Autodesk Inventor part; units mm, degrees
(part 3 of 3)
  line L665 (5.8356, -14.9844) -> (7.0568, -17.6988)
  line L666 (7.0568, -17.6988) -> (8.2692, -14.9844)
  line L667 (8.2692, -14.9844) -> (9.8603, -14.9844)
  line L668 (9.8603, -14.9844) -> (9.8603, -20.4844)
  spline S503 degree 2 poles (14.9057, -18.4119) (14.9057, -19.437) (13.787, -20.6137) (12.7663, -20.6137) knots 0 0 0 1 2 2 2
  spline S504 degree 2 poles (12.7663, -20.6137) (11.7501, -20.6137) (10.6225, -19.437) (10.6225, -18.4119) knots 0 0 0 1 2 2 2
  spline S505 degree 2 poles (10.6225, -18.4119) (10.6225, -17.3779) (11.7501, -16.2057) (12.7663, -16.2057) knots 0 0 0 1 2 2 2
  spline S506 degree 2 poles (12.7663, -16.2057) (13.7825, -16.2057) (14.9057, -17.3823) (14.9057, -18.4119) knots 0 0 0 1 2 2 2
  spline S507 degree 2 poles (13.582, -18.4208) (13.582, -18.0509) (13.4616, -17.5562) (13.3547, -17.4091) knots 0 0 0 1 2 2 2
  spline S508 degree 2 poles (13.3547, -17.4091) (13.2388, -17.2531) (12.9491, -17.1327) (12.7663, -17.1327) knots 0 0 0 1 2 2 2
  spline S509 degree 2 poles (12.7663, -17.1327) (12.588, -17.1327) (12.3073, -17.2397) (12.1914, -17.3912) knots 0 0 0 1 2 2 2
  spline S510 degree 2 poles (12.1914, -17.3912) (12.0799, -17.5339) (11.9462, -18.0375) (11.9462, -18.4208) knots 0 0 0 1 2 2 2
  spline S511 degree 2 poles (11.9462, -18.4208) (11.9462, -18.7997) (12.071, -19.2677) (12.1735, -19.4103) knots 0 0 0 1 2 2 2
  spline S512 degree 2 poles (12.1735, -19.4103) (12.2761, -19.5529) (12.588, -19.6866) (12.7752, -19.6866) knots 0 0 0 1 2 2 2
  spline S513 degree 2 poles (12.7752, -19.6866) (12.9312, -19.6866) (13.2521, -19.5529) (13.3502, -19.4192) knots 0 0 0 1 2 2 2
  spline S514 degree 2 poles (13.3502, -19.4192) (13.4616, -19.2632) (13.582, -18.813) (13.582, -18.4208) knots 0 0 0 1 2 2 2
  spline S515 degree 2 poles (16.8534, -20.5959) (16.3988, -20.5959) (15.5832, -20.3953) (15.3158, -20.2616) knots 0 0 0 1 2 2 2
  line L669 (15.3158, -20.2616) -> (15.3158, -19.1696)
  line L670 (15.3158, -19.1696) -> (15.4227, -19.1696)
  spline S516 degree 2 poles (15.4227, -19.1696) (15.5163, -19.2409) (15.7526, -19.4103) (15.962, -19.5039) knots 0 0 0 1 2 2 2
  spline S517 degree 2 poles (15.962, -19.5039) (16.1448, -19.5886) (16.5949, -19.7089) (16.8624, -19.7089) knots 0 0 0 1 2 2 2
  spline S518 degree 2 poles (16.8624, -19.7089) (17.1342, -19.7089) (17.5532, -19.5395) (17.5532, -19.3568) knots 0 0 0 1 2 2 2
  spline S519 degree 2 poles (17.5532, -19.3568) (17.5532, -19.2142) (17.3615, -19.0626) (17.0852, -19.0002) knots 0 0 0 1 2 2 2
  spline S520 degree 2 poles (17.0852, -19.0002) (16.9381, -18.9601) (16.488, -18.8754) (16.3141, -18.822) knots 0 0 0 1 2 2 2
  spline S521 degree 2 poles (16.3141, -18.822) (15.8239, -18.6704) (15.3336, -18.0776) (15.3336, -17.5918) knots 0 0 0 1 2 2 2
  spline S522 degree 2 poles (15.3336, -17.5918) (15.3336, -17.3155) (15.5876, -16.8252) (15.8372, -16.6335) knots 0 0 0 1 2 2 2
  spline S523 degree 2 poles (15.8372, -16.6335) (16.0824, -16.4463) (16.8089, -16.2235) (17.268, -16.2235) knots 0 0 0 1 2 2 2
  spline S524 degree 2 poles (17.268, -16.2235) (17.7047, -16.2235) (18.4357, -16.3973) (18.6853, -16.5177) knots 0 0 0 1 2 2 2
  line L671 (18.6853, -16.5177) -> (18.6853, -17.5695)
  line L672 (18.6853, -17.5695) -> (18.5828, -17.5695)
  spline S525 degree 2 poles (18.5828, -17.5695) (18.5159, -17.516) (18.2262, -17.3422) (18.0925, -17.2798) knots 0 0 0 1 2 2 2
  spline S526 degree 2 poles (18.0925, -17.2798) (17.9276, -17.2085) (17.5265, -17.1104) (17.317, -17.1104) knots 0 0 0 1 2 2 2
  spline S527 degree 2 poles (17.317, -17.1104) (17.0362, -17.1104) (16.6484, -17.3021) (16.6484, -17.4581) knots 0 0 0 1 2 2 2
  spline S528 degree 2 poles (16.6484, -17.4581) (16.6484, -17.6007) (16.8401, -17.7612) (17.161, -17.8414) knots 0 0 0 1 2 2 2
  spline S529 degree 2 poles (17.161, -17.8414) (17.3259, -17.8815) (17.7582, -17.9573) (17.9588, -18.0241) knots 0 0 0 1 2 2 2
  spline S530 degree 2 poles (17.9588, -18.0241) (18.4045, -18.1668) (18.868, -18.7239) (18.868, -19.1874) knots 0 0 0 1 2 2 2
  spline S531 degree 2 poles (18.868, -19.1874) (18.868, -19.4771) (18.5962, -20.0075) (18.3421, -20.1858) knots 0 0 0 1 2 2 2
  spline S532 degree 2 poles (18.3421, -20.1858) (18.0791, -20.3819) (17.3571, -20.5959) (16.8534, -20.5959) knots 0 0 0 1 2 2 2
  spline S533 degree 2 poles (21.0698, -20.5647) (20.2809, -20.5647) (19.5589, -19.9139) (19.5589, -19.1741) knots 0 0 0 1 2 2 2
  line L673 (19.5589, -19.1741) -> (19.5589, -17.2352)
  line L674 (19.5589, -17.2352) -> (19.0641, -17.2352)
  line L675 (19.0641, -17.2352) -> (19.0641, -16.3349)
  line L676 (19.0641, -16.3349) -> (19.5589, -16.3349)
  line L677 (19.5589, -16.3349) -> (19.5589, -15.1493)
  line L678 (19.5589, -15.1493) -> (20.8514, -15.1493)
  line L679 (20.8514, -15.1493) -> (20.8514, -16.3349)
  line L680 (20.8514, -16.3349) -> (22.0994, -16.3349)
  line L681 (22.0994, -16.3349) -> (22.0994, -17.2352)
  line L682 (22.0994, -17.2352) -> (20.8514, -17.2352)
  line L683 (20.8514, -17.2352) -> (20.8514, -18.7105)
  spline S534 degree 2 poles (20.8514, -18.7105) (20.8514, -18.9289) (20.8603, -19.2543) (20.9138, -19.3835) knots 0 0 0 1 2 2 2
  spline S535 degree 2 poles (20.9138, -19.3835) (20.9673, -19.5128) (21.2303, -19.6643) (21.4799, -19.6643) knots 0 0 0 1 2 2 2
  spline S536 degree 2 poles (21.4799, -19.6643) (21.5868, -19.6643) (21.9211, -19.5752) (21.988, -19.5395) knots 0 0 0 1 2 2 2
  line L684 (21.988, -19.5395) -> (22.0994, -19.5395)
  line L685 (22.0994, -19.5395) -> (22.0994, -20.4488)
  spline S537 degree 2 poles (22.0994, -20.4488) (21.8899, -20.5023) (21.4175, -20.5647) (21.0698, -20.5647) knots 0 0 0 1 2 2 2
  spline S538 degree 2 poles (26.6055, -18.4119) (26.6055, -19.437) (25.4868, -20.6137) (24.4661, -20.6137) knots 0 0 0 1 2 2 2
  spline S539 degree 2 poles (24.4661, -20.6137) (23.4499, -20.6137) (22.3222, -19.437) (22.3222, -18.4119) knots 0 0 0 1 2 2 2
  spline S540 degree 2 poles (22.3222, -18.4119) (22.3222, -17.3779) (23.4499, -16.2057) (24.4661, -16.2057) knots 0 0 0 1 2 2 2
  spline S541 degree 2 poles (24.4661, -16.2057) (25.4823, -16.2057) (26.6055, -17.3823) (26.6055, -18.4119) knots 0 0 0 1 2 2 2
  spline S542 degree 2 poles (25.2817, -18.4208) (25.2817, -18.0509) (25.1614, -17.5562) (25.0544, -17.4091) knots 0 0 0 1 2 2 2
  spline S543 degree 2 poles (25.0544, -17.4091) (24.9385, -17.2531) (24.6488, -17.1327) (24.4661, -17.1327) knots 0 0 0 1 2 2 2
  spline S544 degree 2 poles (24.4661, -17.1327) (24.2878, -17.1327) (24.007, -17.2397) (23.8911, -17.3912) knots 0 0 0 1 2 2 2
  spline S545 degree 2 poles (23.8911, -17.3912) (23.7797, -17.5339) (23.646, -18.0375) (23.646, -18.4208) knots 0 0 0 1 2 2 2
  spline S546 degree 2 poles (23.646, -18.4208) (23.646, -18.7997) (23.7708, -19.2677) (23.8733, -19.4103) knots 0 0 0 1 2 2 2
  spline S547 degree 2 poles (23.8733, -19.4103) (23.9758, -19.5529) (24.2878, -19.6866) (24.475, -19.6866) knots 0 0 0 1 2 2 2
  spline S548 degree 2 poles (24.475, -19.6866) (24.631, -19.6866) (24.9519, -19.5529) (25.05, -19.4192) knots 0 0 0 1 2 2 2
  spline S549 degree 2 poles (25.05, -19.4192) (25.1614, -19.2632) (25.2817, -18.813) (25.2817, -18.4208) knots 0 0 0 1 2 2 2
  line L686 (33.4738, -16.3349) -> (32.2615, -20.4844)
  line L687 (32.2615, -20.4844) -> (30.8887, -20.4844)
  line L688 (30.8887, -20.4844) -> (30.1577, -17.8013)
  line L689 (30.1577, -17.8013) -> (29.4268, -20.4844)
  line L690 (29.4268, -20.4844) -> (28.054, -20.4844)
  line L691 (28.054, -20.4844) -> (26.8506, -16.3349)
  line L692 (26.8506, -16.3349) -> (28.21, -16.3349)
  line L693 (28.21, -16.3349) -> (28.8474, -19.0805)
  line L694 (28.8474, -19.0805) -> (29.6318, -16.3349)
  line L695 (29.6318, -16.3349) -> (30.7773, -16.3349)
  line L696 (30.7773, -16.3349) -> (31.5171, -19.0805)
  line L697 (31.5171, -19.0805) -> (32.1456, -16.3349)
  line L698 (32.1456, -16.3349) -> (33.4738, -16.3349)
  spline S550 degree 2 poles (35.2833, -20.5959) (34.8287, -20.5959) (34.0131, -20.3953) (33.7457, -20.2616) knots 0 0 0 1 2 2 2
  line L699 (33.7457, -20.2616) -> (33.7457, -19.1696)
  line L700 (33.7457, -19.1696) -> (33.8526, -19.1696)
  spline S551 degree 2 poles (33.8526, -19.1696) (33.9462, -19.2409) (34.1825, -19.4103) (34.3919, -19.5039) knots 0 0 0 1 2 2 2
  spline S552 degree 2 poles (34.3919, -19.5039) (34.5747, -19.5886) (35.0248, -19.7089) (35.2923, -19.7089) knots 0 0 0 1 2 2 2
  spline S553 degree 2 poles (35.2923, -19.7089) (35.5641, -19.7089) (35.9831, -19.5395) (35.9831, -19.3568) knots 0 0 0 1 2 2 2
  spline S554 degree 2 poles (35.9831, -19.3568) (35.9831, -19.2142) (35.7915, -19.0626) (35.5151, -19.0002) knots 0 0 0 1 2 2 2
  spline S555 degree 2 poles (35.5151, -19.0002) (35.368, -18.9601) (34.9179, -18.8754) (34.744, -18.822) knots 0 0 0 1 2 2 2
  spline S556 degree 2 poles (34.744, -18.822) (34.2538, -18.6704) (33.7635, -18.0776) (33.7635, -17.5918) knots 0 0 0 1 2 2 2
  spline S557 degree 2 poles (33.7635, -17.5918) (33.7635, -17.3155) (34.0175, -16.8252) (34.2671, -16.6335) knots 0 0 0 1 2 2 2
  spline S558 degree 2 poles (34.2671, -16.6335) (34.5123, -16.4463) (35.2388, -16.2235) (35.6979, -16.2235) knots 0 0 0 1 2 2 2
  spline S559 degree 2 poles (35.6979, -16.2235) (36.1346, -16.2235) (36.8656, -16.3973) (37.1152, -16.5177) knots 0 0 0 1 2 2 2
  line L701 (37.1152, -16.5177) -> (37.1152, -17.5695)
  line L702 (37.1152, -17.5695) -> (37.0127, -17.5695)
  spline S560 degree 2 poles (37.0127, -17.5695) (36.9458, -17.516) (36.6561, -17.3422) (36.5224, -17.2798) knots 0 0 0 1 2 2 2
  spline S561 degree 2 poles (36.5224, -17.2798) (36.3575, -17.2085) (35.9564, -17.1104) (35.7469, -17.1104) knots 0 0 0 1 2 2 2
  spline S562 degree 2 poles (35.7469, -17.1104) (35.4661, -17.1104) (35.0783, -17.3021) (35.0783, -17.4581) knots 0 0 0 1 2 2 2
  spline S563 degree 2 poles (35.0783, -17.4581) (35.0783, -17.6007) (35.27, -17.7612) (35.5909, -17.8414) knots 0 0 0 1 2 2 2
  spline S564 degree 2 poles (35.5909, -17.8414) (35.7558, -17.8815) (36.1881, -17.9573) (36.3887, -18.0241) knots 0 0 0 1 2 2 2
  spline S565 degree 2 poles (36.3887, -18.0241) (36.8344, -18.1668) (37.2979, -18.7239) (37.2979, -19.1874) knots 0 0 0 1 2 2 2
  spline S566 degree 2 poles (37.2979, -19.1874) (37.2979, -19.4771) (37.0261, -20.0075) (36.772, -20.1858) knots 0 0 0 1 2 2 2
  spline S567 degree 2 poles (36.772, -20.1858) (36.509, -20.3819) (35.787, -20.5959) (35.2833, -20.5959) knots 0 0 0 1 2 2 2
  line L703 (42.067, -20.4844) -> (40.5293, -20.4844)
  line L704 (40.5293, -20.4844) -> (39.4061, -18.6838)
  line L705 (39.4061, -18.6838) -> (39.2056, -18.9512)
  line L706 (39.2056, -18.9512) -> (39.2056, -20.4844)
  line L707 (39.2056, -20.4844) -> (37.913, -20.4844)
  line L708 (37.913, -20.4844) -> (37.913, -14.7393)
  line L709 (37.913, -14.7393) -> (39.2056, -14.7393)
  line L710 (39.2056, -14.7393) -> (39.2056, -17.9573)
  line L711 (39.2056, -17.9573) -> (40.4312, -16.3349)
  line L712 (40.4312, -16.3349) -> (41.96, -16.3349)
  line L713 (41.96, -16.3349) -> (40.507, -18.1222)
  line L714 (40.507, -18.1222) -> (42.067, -20.4844)
  line L715 (43.7651, -20.4844) -> (42.4726, -20.4844)
  line L716 (42.4726, -20.4844) -> (42.4726, -16.3349)
  line L717 (42.4726, -16.3349) -> (43.7651, -16.3349)
  line L718 (43.7651, -16.3349) -> (43.7651, -20.4844)
  line L719 (43.8052, -15.7421) -> (42.4369, -15.7421)
  line L720 (42.4369, -15.7421) -> (42.4369, -14.7348)
  line L721 (42.4369, -14.7348) -> (43.8052, -14.7348)
  line L722 (43.8052, -14.7348) -> (43.8052, -15.7421)
  spline S568 degree 2 poles (46.8806, -20.5959) (45.7039, -20.5959) (44.4515, -19.4727) (44.4515, -18.4342) knots 0 0 0 1 2 2 2
  spline S569 degree 2 poles (44.4515, -18.4342) (44.4515, -17.418) (45.6192, -16.2057) (46.6711, -16.2057) knots 0 0 0 1 2 2 2
  spline S570 degree 2 poles (46.6711, -16.2057) (47.6205, -16.2057) (48.5832, -17.2352) (48.5832, -18.1891) knots 0 0 0 1 2 2 2
  line L723 (48.5832, -18.1891) -> (48.5832, -18.657)
  line L724 (48.5832, -18.657) -> (45.744, -18.657)
  spline S571 degree 2 poles (45.744, -18.657) (45.7619, -18.9468) (45.9714, -19.3301) (46.1407, -19.4459) knots 0 0 0 1 2 2 2
  spline S572 degree 2 poles (46.1407, -19.4459) (46.3056, -19.5618) (46.7513, -19.6599) (47.0143, -19.6599) knots 0 0 0 1 2 2 2
  spline S573 degree 2 poles (47.0143, -19.6599) (47.2372, -19.6599) (47.6739, -19.5618) (47.8567, -19.4771) knots 0 0 0 1 2 2 2
  spline S574 degree 2 poles (47.8567, -19.4771) (48.0171, -19.4103) (48.2846, -19.2454) (48.3692, -19.183) knots 0 0 0 1 2 2 2
  line L725 (48.3692, -19.183) -> (48.5074, -19.183)
  line L726 (48.5074, -19.183) -> (48.5074, -20.2527)
  spline S575 degree 2 poles (48.5074, -20.2527) (48.347, -20.3151) (48.0885, -20.422) (47.8567, -20.4755) knots 0 0 0 1 2 2 2
  spline S576 degree 2 poles (47.8567, -20.4755) (47.6472, -20.5335) (47.2015, -20.5959) (46.8806, -20.5959) knots 0 0 0 1 2 2 2
  spline S577 degree 2 poles (47.3085, -17.8771) (47.2996, -17.467) (46.9385, -17.0347) (46.5686, -17.0347) knots 0 0 0 1 2 2 2
  spline S578 degree 2 poles (46.5686, -17.0347) (46.1898, -17.0347) (45.7619, -17.4893) (45.7396, -17.8771) knots 0 0 0 1 2 2 2
  line L727 (45.7396, -17.8771) -> (47.3085, -17.8771)
  spline S579 degree 2 poles (53.018, -20.0075) (53.018, -20.5825) (52.6837, -21.3892) (52.3984, -21.6121) knots 0 0 0 1 2 2 2
  spline S580 degree 2 poles (52.3984, -21.6121) (52.1087, -21.8394) (51.3064, -22.0444) (50.8162, -22.0444) knots 0 0 0 1 2 2 2
  spline S581 degree 2 poles (50.8162, -22.0444) (50.4017, -22.0444) (49.6573, -21.9374) (49.3855, -21.8661) knots 0 0 0 1 2 2 2
  line L728 (49.3855, -21.8661) -> (49.3855, -20.8276)
  line L729 (49.3855, -20.8276) -> (49.537, -20.8276)
  spline S582 degree 2 poles (49.537, -20.8276) (49.6306, -20.8633) (49.8936, -20.9524) (50.0273, -20.9881) knots 0 0 0 1 2 2 2
  spline S583 degree 2 poles (50.0273, -20.9881) (50.1877, -21.0282) (50.4908, -21.0817) (50.6468, -21.0817) knots 0 0 0 1 2 2 2
  spline S584 degree 2 poles (50.6468, -21.0817) (50.9766, -21.0817) (51.4134, -20.948) (51.5248, -20.8232) knots 0 0 0 1 2 2 2
  spline S585 degree 2 poles (51.5248, -20.8232) (51.6363, -20.6939) (51.7254, -20.3463) (51.7254, -20.0788) knots 0 0 0 1 2 2 2
  line L730 (51.7254, -20.0788) -> (51.7254, -20.0031)
  spline S586 degree 2 poles (51.7254, -20.0031) (51.507, -20.1947) (50.9365, -20.4265) (50.6334, -20.4265) knots 0 0 0 1 2 2 2
  spline S587 degree 2 poles (50.6334, -20.4265) (49.8267, -20.4265) (48.9531, -19.3791) (48.9531, -18.3049) knots 0 0 0 1 2 2 2
  spline S588 degree 2 poles (48.9531, -18.3049) (48.9531, -17.8191) (49.2205, -17.0436) (49.4612, -16.7717) knots 0 0 0 1 2 2 2
  spline S589 degree 2 poles (49.4612, -16.7717) (49.693, -16.5087) (50.3393, -16.2235) (50.6914, -16.2235) knots 0 0 0 1 2 2 2
  spline S590 degree 2 poles (50.6914, -16.2235) (51.0078, -16.2235) (51.5115, -16.384) (51.7165, -16.5177) knots 0 0 0 1 2 2 2
  line L731 (51.7165, -16.5177) -> (51.7655, -16.3349)
  line L732 (51.7655, -16.3349) -> (53.018, -16.3349)
  line L733 (53.018, -16.3349) -> (53.018, -20.0075)
  line L734 (51.7254, -19.1785) -> (51.7254, -17.2976)
  spline S591 degree 2 poles (51.7254, -17.2976) (51.6318, -17.2531) (51.351, -17.1951) (51.2084, -17.1951) knots 0 0 0 1 2 2 2
  spline S592 degree 2 poles (51.2084, -17.1951) (50.7449, -17.1951) (50.2769, -17.7968) (50.2769, -18.3361) knots 0 0 0 1 2 2 2
  spline S593 degree 2 poles (50.2769, -18.3361) (50.2769, -18.6036) (50.3482, -18.978) (50.4418, -19.1206) knots 0 0 0 1 2 2 2
  spline S594 degree 2 poles (50.4418, -19.1206) (50.5354, -19.2632) (50.834, -19.4058) (51.0658, -19.4058) knots 0 0 0 1 2 2 2
  spline S595 degree 2 poles (51.0658, -19.4058) (51.2396, -19.4058) (51.5739, -19.2855) (51.7254, -19.1785) knots 0 0 0 1 2 2 2
  spline S596 degree 2 poles (57.9876, -18.4119) (57.9876, -19.437) (56.8688, -20.6137) (55.8482, -20.6137) knots 0 0 0 1 2 2 2
  spline S597 degree 2 poles (55.8482, -20.6137) (54.832, -20.6137) (53.7043, -19.437) (53.7043, -18.4119) knots 0 0 0 1 2 2 2
  spline S598 degree 2 poles (53.7043, -18.4119) (53.7043, -17.3779) (54.832, -16.2057) (55.8482, -16.2057) knots 0 0 0 1 2 2 2
  spline S599 degree 2 poles (55.8482, -16.2057) (56.8644, -16.2057) (57.9876, -17.3823) (57.9876, -18.4119) knots 0 0 0 1 2 2 2
  spline S600 degree 2 poles (56.6638, -18.4208) (56.6638, -18.0509) (56.5435, -17.5562) (56.4365, -17.4091) knots 0 0 0 1 2 2 2
  spline S601 degree 2 poles (56.4365, -17.4091) (56.3206, -17.2531) (56.0309, -17.1327) (55.8482, -17.1327) knots 0 0 0 1 2 2 2
  spline S602 degree 2 poles (55.8482, -17.1327) (55.6699, -17.1327) (55.3891, -17.2397) (55.2732, -17.3912) knots 0 0 0 1 2 2 2
  spline S603 degree 2 poles (55.2732, -17.3912) (55.1618, -17.5339) (55.0281, -18.0375) (55.0281, -18.4208) knots 0 0 0 1 2 2 2
  spline S604 degree 2 poles (55.0281, -18.4208) (55.0281, -18.7997) (55.1529, -19.2677) (55.2554, -19.4103) knots 0 0 0 1 2 2 2
  spline S605 degree 2 poles (55.2554, -19.4103) (55.3579, -19.5529) (55.6699, -19.6866) (55.8571, -19.6866) knots 0 0 0 1 2 2 2
  spline S606 degree 2 poles (55.8571, -19.6866) (56.0131, -19.6866) (56.334, -19.5529) (56.4321, -19.4192) knots 0 0 0 1 2 2 2
  spline S607 degree 2 poles (56.4321, -19.4192) (56.5435, -19.2632) (56.6638, -18.813) (56.6638, -18.4208) knots 0 0 0 1 2 2 2
  point P0 (0, 0)
  constraints: 2 other
extrude "Extrusion2" add sketch "Sketch2" along normal blind 0.8
sketch "Sketch3" plane through (0, 1.2, 0) normal (0, 1, 0) x (1, 0, 0)
  line L0 (85, -25) -> (85, 25) projected
  line L1 (-85, 25) -> (-85, -25) projected
  circle A0 centre (-70, 0) radius 1.7
  circle A1 centre (70, 0) radius 1.7
  point P0 (0, 0)
  dimension "d6" = 3.4
  dimension "d7" = 3.4
  dimension "d8" = 15
  dimension "d9" = 15
  constraints: 2 centre point
  measures "d6" diameter of A0
  measures "d7" diameter of A1
  measures "d8" distance from line of A0.centre L1
  measures "d9" distance from line of L0 A1.centre
extrude "Extrusion3" cut sketch "Sketch3" against normal through all
body "Solid1"
